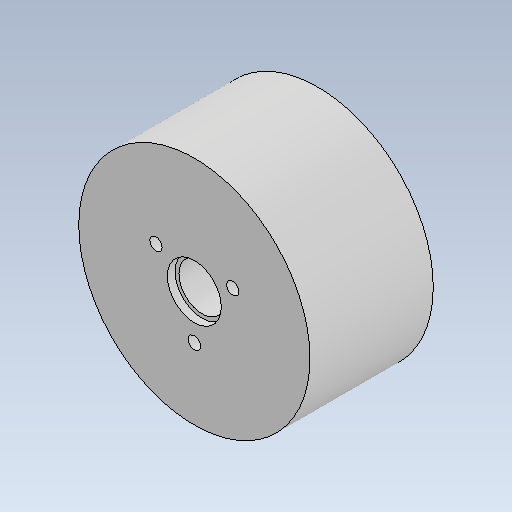
# Autodesk Inventor part: mecanumL
Saved by Autodesk Inventor 2026.1 (Build 301233020, 233B)
## iProperties
Created: 2026-10-09
Part Number: mecanumL
Material: 一般
Document SubType Name: Modeling
Designer: ug_nd
Density: 1 g/cm^3
Appearance: 既定
Author: ug_nd
Autodesk Inventor part; units mm, degrees
ref_plane "YZ Plane" through (0, 0, 0) normal (1, 0, 0) x (0, 1, 0)
ref_plane "XZ Plane" through (0, 0, 0) normal (0, 1, 0) x (-1, 0, 0)
ref_plane "XY Plane" through (0, 0, 0) normal (0, 0, 1) x (1, 0, 0)
sketch "スケッチ1" plane through (0, 0, 0) normal (0, 0, 1) x (1, 0, 0)
  circle A0 centre (0, 0) radius 30
  circle A1 centre (0, 0) radius 6
  dimension "d0" = 12
  dimension "d1" = 60
  constraints: 2 centre point, 2 coincident
  measures "d0" diameter of A1
  measures "d1" diameter of A0
extrude "押し出し1" add sketch "スケッチ1" along normal mid plane 32
sketch "スケッチ3" plane through (0, 0, 16) normal (0, 0, 1) x (1, 0, 0)
  circle A0 centre (0, 0) radius 11.5 construction
  circle A1 centre (-9.9593, 5.75) radius 1.6
  circle A2 centre (0, -11.5) radius 1.6
  circle A3 centre (9.9593, 5.75) radius 1.6
  dimension "d7" = 23
  dimension "d8" = 3.2
  dimension "d11" = 360
  constraints: 3 centre point, 1 coincident, 1 vertical alignment, 10 other
  measures "d8" diameter of A1
extrude "押し出し3" cut sketch "スケッチ3" against normal through all
sketch "スケッチ2" plane through (0, 0, 16) normal (0, 0, 1) x (1, 0, 0)
  circle A0 centre (0, 0) radius 7
  dimension "d4" = 14
  constraints: 1 centre point, 1 coincident
  measures "d4" diameter of A0
extrude "押し出し2" cut sketch "スケッチ2" against normal blind 2
mirror "ミラー1" about plane through (0, 0, 0) normal (0, 0, 1) of "押し出し2"
